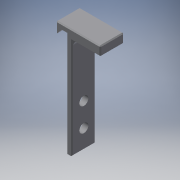
# Autodesk Inventor part: Battery Latch
Saved by Autodesk Inventor 2017 (Build 210142000, 142)
## iProperties
Created: 2015-06-08
Part Number: Battery Latch
Material: Generic
Document SubType Name: Modeling
Designer: Dale
Density: 1 g/cm^3
Appearance: Default
Author: Dale
Autodesk Inventor part; units mm, degrees
ref_plane "YZ Plane" through (0, 0, 0) normal (1, 0, 0) x (0, 1, 0)
ref_plane "XZ Plane" through (0, 0, 0) normal (0, 1, 0) x (-1, 0, 0)
ref_plane "XY Plane" through (0, 0, 0) normal (0, 0, 1) x (1, 0, 0)
sketch "Sketch1" plane through (0, 0, 0) normal (0, 0, 1) x (1, 0, 0)
  line L0 (-2.4, 0) -> (-2.4, 44)
  line L1 (-2.4, 44) -> (-4.7, 44)
  line L2 (-4.7, 44) -> (-6.4, 42)
  line L3 (-6.4, 42) -> (-6.8, 42)
  line L4 (-6.8, 42) -> (-6.8, 46.5)
  line L5 (-6.8, 46.5) -> (12, 46.5)
  line L6 (12, 46.5) -> (12, 42.5)
  line L7 (12, 42.5) -> (0, 42.5)
  line L8 (0, 42.5) -> (0, 0)
  line L9 (0, 0) -> (-2.4, 0)
  dimension "d0" = 44
  dimension "d3" = 2.4
  dimension "d5" = 2.5
  dimension "d6" = 4
  dimension "d7" = 12
  dimension "d19" = 18.8
  dimension "d20" = 0.4
  dimension "d21" = 2
  dimension "d22" = 2.3
  constraints: 20 end point, 4 horizontal, 4 vertical, 1 coincident
  measures "d0" distance of L0.end L0.start
  measures "d3" distance between parallel lines of L8 L0
  measures "d5" distance between parallel lines of L5 L1
  measures "d6" distance between parallel lines of L7 L5
  measures "d7" distance of L6.end L7.end
  measures "d19" distance of L4.end L5.end
  measures "d20" distance of L2.end L3.end
  measures "d21" vertical distance of L1.end L2.end
  measures "d22" distance of L0.end L1.end
extrude "Extrusion1" add sketch "Sketch1" along normal blind 10
sketch "Sketch2" plane through (0, 0, 0) normal (1, 0, 0) x (0, 0, -1)
  circle A0 centre (-5, 8) radius 1.9
  line L0 (0, 0) -> (-10, 0) projected
  line L1 (-10, 0) -> (-10, 42.5) projected
  line L2 (0, 42.5) -> (-10, 42.5) projected
  circle A1 centre (-5, 18) radius 1.9
  dimension "d10" = 3.8
  dimension "d11" = 8
  dimension "d12" = 5
  dimension "d23" = 34.5
  dimension "d26" = 10
  constraints: 2 centre point, 1 vertical, 2 other
  measures "d10" diameter of A0
  measures "d11" distance from line of L0 A0.centre
  measures "d12" distance from line of A0.centre L1
  measures "d23" distance from line of A0.centre L2
  measures "d26" distance of A0.centre A1.centre
extrude "Extrusion3" cut sketch "Sketch2" against normal through all
chamfer "Chamfer1" distance 0.4 angle 45 19 edges at (0, 21.25, 10) (0, 0, 5) (0, 21.25, 0) (6, 42.5, 0) (6, 42.5, 10) (12, 42.5, 5) (12, 46.5, 5) (12, 44.5, 10) (12, 44.5, 0) (-6.8, 46.5, 5) (2.6, 46.5, 10) (2.6, 46.5, 0) (-6.8, 44.25, 0) (-6.8, 44.25, 10) (-2.4, 22, 0) (-2.4, 0, 5) (-2.4, 22, 10) (-3.55, 44, 10) (-3.55, 44, 0)
fillet "Fillet1" radius 2 1 edges at (0, 42.5, 5)
body "Solid1"
